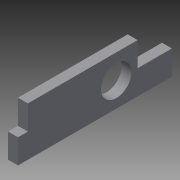
# Autodesk Inventor part: body-side2
Saved by Autodesk Inventor 2013 (Build 170138000, 138)
## iProperties
Created: 2012-09-08
Part Number: body-side2
Material: Generic
Document SubType Name: Modeling
Designer: frankenteddy
Density: 1 g/cm^3
Author: frankenteddy
Autodesk Inventor part; units mm, degrees
ref_plane "YZ Plane" through (0, 0, 0) normal (1, 0, 0) x (0, 1, 0)
ref_plane "XZ Plane" through (0, 0, 0) normal (0, 1, 0) x (-1, 0, 0)
ref_plane "XY Plane" through (0, 0, 0) normal (0, 0, 1) x (1, 0, 0)
sketch "Sketch1" plane through (0, 0, 0) normal (1, 0, 0) x (0, 1, 0)
  line L0 (-92.7646, -8.503) -> (-89.7646, -8.503)
  line L1 (-89.7646, -8.503) -> (-89.7646, -11.753)
  line L2 (-89.7646, -11.753) -> (-92.7646, -11.753)
  line L3 (-92.7646, -11.753) -> (-92.7646, -8.503)
  line L4 (-92.7646, -21.6527) -> (-89.7646, -21.6527)
  line L5 (-89.7646, -21.6527) -> (-89.7646, -21.7527)
  line L6 (-89.7646, -21.7527) -> (-92.7646, -21.7527)
  line L7 (-92.7646, -21.7527) -> (-92.7646, -21.6527)
  line L8 (-56.4516, 8.2437) -> (-59.7016, 8.2437)
  line L9 (-59.7016, 8.2437) -> (-59.7016, 16.2437)
  line L10 (-59.7016, 16.2437) -> (-56.4516, 16.2437)
  line L11 (-56.4516, 16.2437) -> (-56.4516, 8.2437)
  line L12 (-34.4516, 24.2437) -> (-34.4516, 8.2437) construction
  line L13 (-12.4516, 8.2437) -> (-9.2016, 8.2437)
  line L14 (-9.2016, 8.2437) -> (-9.2016, 16.2437)
  line L15 (-9.2016, 16.2437) -> (-12.4516, 16.2437)
  line L16 (-12.4516, 16.2437) -> (-12.4516, 8.2437)
  circle A0 centre (-27.4516, 16.2437) radius 5
  line L17 (-12.4516, 8.2437) -> (-20.4516, 8.2437)
  line L18 (-20.4516, 8.2437) -> (-20.4516, 16.2437)
  line L19 (-20.4516, 16.2437) -> (-12.4516, 16.2437)
  line L20 (-12.4516, 16.2437) -> (-12.4516, 8.2437)
  line L21 (-20.4516, 8.2437) -> (-56.4516, 8.2437)
  line L22 (-56.4516, 8.2437) -> (-56.4516, 24.2437)
  line L23 (-56.4516, 24.2437) -> (-20.4516, 24.2437)
  line L24 (-20.4516, 24.2437) -> (-20.4516, 8.2437)
  point P0 (0, 0)
  dimension "d0" = 3
  dimension "mat" = 3.25
  dimension "d2" = 3
  dimension "kerf" = 0.1
  dimension "d27" = 3.25
  dimension "d28" = 8
  dimension "d29" = 10
  dimension "d34" = 2
  dimension "d35" = 8
  dimension "d38" = 36
  constraints: 50 end point, 10 parallel, 5 horizontal, 5 perpendicular, 3 symmetric about line, 1 centre point, 1 collinear
  measures "d0" distance of L1.end L2.end
  measures "mat" distance of L0.end L1.end
  measures "d2" distance of L5.end L6.end
  measures "kerf" distance of L4.end L5.end
  measures "d27" distance of L9.end L10.end
  measures "d28" distance of L8.end L9.end
  measures "d29" diameter of A0
  measures "d34" distance edge to line of A0 L18
  measures "d35" distance of L18.end L19.end
  measures "d38" distance of L22.end L23.end
extrude "Extrusion5" add sketch "Sketch1" along normal blind 3.25 contours L8 L9 L10 L11 | L11 L22 L23 L24 L18 L21 | L18 L19 L16 L17 | L16 L15 L14 L13
equation "\"d27\" = mat"
equation "\"d36\" = mat"
body "Solid3"
